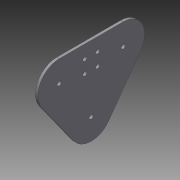
# Autodesk Inventor part: Arm_Base-SquareBar-Rev3
Saved by Autodesk Inventor 2015 (Build 190159000, 159)
## iProperties
Created: 2017-01-08
Part Number: Arm_Base-SquareBar-Rev3
Material: Generic
Document SubType Name: Modeling
Designer: Guy
Density: 1 g/cm^3
Appearance: Default
Author: Guy
Autodesk Inventor part; units mm, degrees
ref_plane "YZ Plane" through (0, 0, 0) normal (1, 0, 0) x (0, 1, 0)
ref_plane "XZ Plane" through (0, 0, 0) normal (0, 1, 0) x (-1, 0, 0)
ref_plane "XY Plane" through (0, 0, 0) normal (0, 0, 1) x (1, 0, 0)
sketch "Sketch1" plane through (0, 0, 0) normal (1, 0, 0) x (0, 1, 0)
  circle A0 centre (105, 75) radius 50
  circle A1 centre (105, -75) radius 50
  circle A2 centre (0, 0) radius 50
  line L0 (75.9381, 115.6867) -> (-29.0619, 40.6867)
  line L1 (-29.0619, -40.6867) -> (75.9381, -115.6867)
  line L2 (155, -75) -> (155, 75)
  dimension "d0" = 150
  dimension "d1" = 105
  dimension "d2" = 105
  dimension "d3" = 75
  dimension "d4" = 100
  dimension "d5" = 100
  dimension "d6" = 100
  constraints: 6 end point, 6 point on circle, 6 tangent, 3 centre point, 1 coincident
  measures "d0" distance of A0.centre A1.centre
  measures "d1" horizontal distance of point (0, 0) A0.centre
  measures "d2" horizontal distance of point (0, 0) A1.centre
  measures "d3" vertical distance of point (0, 0) A1.centre
  measures "d4" diameter of A0
  measures "d5" diameter of A1
  measures "d6" diameter of A2
extrude "Extrusion1" add sketch "Sketch1" along normal blind 6
sketch "Sketch2" plane through (6, 0, 0) normal (1, 0, 0) x (0, 0, -1)
  circle A0 centre (-75, 105) radius 5
  circle A1 centre (75, 105) radius 5
  circle A2 centre (0, 0) radius 5
  arc A3 (-40.6867, -29.0619) -> (40.6867, -29.0619) centre (0, 0) ccw projected
  line L0 (40.6867, -29.0619) -> (115.6867, 75.9381) projected
  arc A4 (115.6867, 75.9381) -> (75, 155) centre (75, 105) ccw projected
  line L1 (75, 155) -> (-75, 155) projected
  arc A5 (-75, 155) -> (-115.6867, 75.9381) centre (-75, 105) ccw projected
  line L2 (-115.6867, 75.9381) -> (-40.6867, -29.0619) projected
  dimension "d9" = 10
  dimension "d10" = 10
  dimension "d11" = 10
  constraints: 3 centre point, 3 coincident
  measures "d9" diameter of A0
  measures "d10" diameter of A1
  measures "d11" diameter of A2
extrude "Extrusion2" cut sketch "Sketch2" against normal up to next contours A0 | A1 | A2
sketch "Sketch3" plane through (6, 0, 0) normal (1, 0, 0) x (0, 0, -1)
  circle A0 centre (75, 105) radius 5 projected
  circle A1 centre (-75, 105) radius 5 projected
  circle A2 centre (0, 0) radius 5 projected
  arc A3 (-40.6867, -29.0619) -> (40.6867, -29.0619) centre (0, 0) ccw projected
  line L0 (40.6867, -29.0619) -> (115.6867, 75.9381) projected
  arc A4 (115.6867, 75.9381) -> (75, 155) centre (75, 105) ccw projected
  line L1 (75, 155) -> (-75, 155) projected
  arc A5 (-75, 155) -> (-115.6867, 75.9381) centre (-75, 105) ccw projected
  line L2 (-115.6867, 75.9381) -> (-40.6867, -29.0619) projected
  circle A6 centre (-15, 95) radius 5
  circle A7 centre (15, 95) radius 5
  circle A8 centre (15, 125) radius 5
  circle A9 centre (-15, 125) radius 5
  dimension "d14" = 10
  dimension "d15" = 10
  dimension "d16" = 10
  dimension "d17" = 10
  dimension "d18" = 30
  dimension "d19" = 30
  dimension "d20" = 30
  dimension "d21" = 30
  dimension "d22" = 30
  dimension "d23" = 15
  dimension "d24" = 15
  dimension "d25" = 30
  constraints: 4 centre point
  measures "d14" diameter of A8
  measures "d15" diameter of A9
  measures "d16" diameter of A7
  measures "d17" diameter of A6
  measures "d18" distance of A8.centre A9.centre
  measures "d19" distance of A6.centre A7.centre
  measures "d20" distance of A7.centre A8.centre
  measures "d21" distance of A6.centre A9.centre
  measures "d22" distance from line of L1 A9.centre
  measures "d23" horizontal distance of point (0, 0) A7.centre
  measures "d24" horizontal distance of A2.centre A8.centre
  measures "d25" distance from line of L1 A8.centre
extrude "Extrusion3" cut sketch "Sketch3" against normal blind 6 contours A6 | A7 | A8 | A9
body "Solid1"
